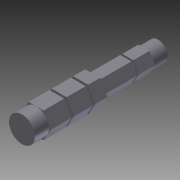
# Autodesk Inventor part: shaft - step down No. 1 - 0.5 hex
Saved by Autodesk Inventor 2012 (Build 160160000, 160)
## iProperties
Created: 2012-02-05
Part Number: shaft - step down No. 1 - 0.5 hex
Material: Steel
Document SubType Name: Modeling
Designer: Antonella Wilby
Mass: 56.1486 g
Surface Area: 25.2544 cm^2
Volume: 7.15269 cm^3
Density: 7.85 g/cm^3
Author: Antonella Wilby
Autodesk Inventor part; units mm, degrees
sketch "Sketch1" plane through (0, 0, 0) normal (0, 0, 1) x (1, 0, 0)
  line L0 (-10.3063, 0) -> (10.3063, 0) projected
  line L1 (0, -8.9256) -> (0, 8.9256) projected
  line L2 (3.6808, 6.3754) -> (7.3617, 0)
  line L3 (7.3617, 0) -> (3.6808, -6.3754)
  line L4 (3.6808, -6.3754) -> (-3.6808, -6.3754)
  line L5 (-3.6808, -6.3754) -> (-7.3617, 0)
  line L6 (-7.3617, 0) -> (-3.6808, 6.3754)
  line L7 (-3.6808, 6.3754) -> (3.6808, 6.3754)
  point P0 (0, 0)
  point P1 (0, 0)
  point P2 (0, 6.3754)
  dimension "d0" = 12.7508
  constraints: 12 end point, 1 coincident, 1 midpoint, 1 vertical alignment, 13 other
  measures "d0" distance between parallel lines of L7 L4
extrude "Base" add sketch "Sketch1" along normal mid plane 67.3354
sketch "Sketch2" plane through (0, 0, 33.6677) normal (0, 0, 1) x (1, 0, 0)
  line L0 (7.3617, 0) -> (3.6808, -6.3754) projected
  line L1 (3.6808, 6.3754) -> (7.3617, 0) projected
  line L2 (-3.6808, 6.3754) -> (3.6808, 6.3754) projected
  line L3 (-7.3617, 0) -> (-3.6808, 6.3754) projected
  line L4 (-3.6808, -6.3754) -> (-7.3617, 0) projected
  line L5 (3.6808, -6.3754) -> (-3.6808, -6.3754) projected
  circle A0 centre (0, 0) radius 6.3754
  constraints: 1 centre point, 1 coincident, 1 tangent
extrude "Bearing Fit" cut sketch "Sketch2" against normal blind 6.985 contours L0 A0 L1 | L0 L5 A0 | A0 L2 L1 | L5 L4 A0 | A0 L3 L2 | L4 L3 A0
mirror "Mirror1" about plane through (0, 0, 0) normal (0, 0, 1) of "Bearing Fit"
sketch "Sketch4" plane through (0, 0, -33.6677) normal (0, 0, -1) x (-1, 0, 0)
  circle A0 centre (0, 0) radius 6.3754 projected
  circle A1 centre (0, 0) radius 4.7625
  dimension "d7" = 9.525
  constraints: 1 centre point, 1 coincident
  measures "d7" diameter of A1
extrude "Extrusion4" cut sketch "Sketch4" against normal up to surface (6.985 mm away)
sketch "Sketch5" plane through (3.6808, 6.3754, -26.6827) normal (0, 0, -1) x (-1, 0, 0)
  line L0 (7.3617, 0) -> (11.0425, -6.3754) projected
  line L1 (0, 0) -> (7.3617, 0) projected
  line L2 (-3.6808, -6.3754) -> (0, 0) projected
  line L3 (0, -12.7508) -> (-3.6808, -6.3754) projected
  line L4 (7.3617, -12.7508) -> (0, -12.7508) projected
  line L5 (11.0425, -6.3754) -> (7.3617, -12.7508) projected
  line L6 (6.4305, -1.6129) -> (9.1801, -6.3754)
  line L7 (9.1801, -6.3754) -> (6.4305, -11.1379)
  line L8 (6.4305, -11.1379) -> (0.9312, -11.1379)
  line L9 (0.9312, -11.1379) -> (-1.8184, -6.3754)
  line L10 (-1.8184, -6.3754) -> (0.9312, -1.6129)
  line L11 (0.9312, -1.6129) -> (6.4305, -1.6129)
  dimension "d10" = 9.525
  constraints: 12 end point, 5 other
  measures "d10" distance between parallel lines of L11 L8
extrude ".375 step down" cut sketch "Sketch5" against normal blind 25.4
ref_plane "Work Plane1" through (0, 0, 15.2527) normal (0, 0, 1) x (1, 0, 0)
sketch "Sketch6" plane through (0, 0, 15.2527) normal (0, 0, 1) x (1, 0, 0)
  line L0 (-3.6808, 6.3754) -> (0, 6.3754) projected
  line L1 (-5.5213, 3.1877) -> (-3.6808, 6.3754) projected
  line L2 (3.6808, 6.3754) -> (5.5213, 3.1877) projected
  line L3 (0, 6.3754) -> (3.6808, 6.3754) projected
  line L4 (5.5213, 3.1877) -> (7.3617, 0) projected
  line L5 (7.3617, 0) -> (5.5213, -3.1877) projected
  line L6 (5.5213, -3.1877) -> (3.6808, -6.3754) projected
  line L7 (0, -6.3754) -> (-3.6808, -6.3754) projected
  line L8 (-3.6808, -6.3754) -> (-5.5213, -3.1877) projected
  line L9 (3.6808, -6.3754) -> (0, -6.3754) projected
  line L10 (-7.3617, 0) -> (-5.5213, 3.1877) projected
  line L11 (-5.5213, -3.1877) -> (-7.3617, 0) projected
  circle A0 centre (0, 0) radius 5.0292
  point P0 (0, 0)
  dimension "d14" = 10.0584
  constraints: 1 centre point, 1 coincident
  measures "d14" diameter of A0
extrude "Extrusion6" cut sketch "Sketch6" along normal blind 1.1684
ref_plane "Work Plane2" through (0, 0, 5.7785) normal (0, 0, 1) x (1, 0, 0)
sketch "Sketch7" plane through (0, 0, 5.7785) normal (0, 0, 1) x (1, 0, 0)
  line L0 (0, 6.3754) -> (3.6808, 6.3754) projected
  line L1 (3.6808, 6.3754) -> (5.5213, 3.1877) projected
  line L2 (5.5213, 3.1877) -> (7.3617, 0) projected
  line L3 (7.3617, 0) -> (5.5213, -3.1877) projected
  line L4 (5.5213, -3.1877) -> (3.6808, -6.3754) projected
  line L5 (3.6808, -6.3754) -> (0, -6.3754) projected
  line L6 (0, -6.3754) -> (-3.6808, -6.3754) projected
  line L7 (-3.6808, -6.3754) -> (-5.5213, -3.1877) projected
  line L8 (-7.3617, 0) -> (-5.5213, 3.1877) projected
  line L9 (-5.5213, 3.1877) -> (-3.6808, 6.3754) projected
  line L10 (-3.6808, 6.3754) -> (0, 6.3754) projected
  circle A0 centre (0, 0) radius 5.0292
  circle A1 centre (0, 0) radius 7.3617
  point P0 (0, 0)
  dimension "d18" = 10.0584
  constraints: 2 coincident, 1 centre point, 3 other
  measures "d18" diameter of A0
extrude "Extrusion7" cut sketch "Sketch7" against normal blind 1.1684
ref_plane "Work Plane3" through (0, 0, -18.7071) normal (0, 0, 1) x (1, 0, 0)
sketch "Sketch8" plane through (0, 0, -18.7071) normal (0, 0, 1) x (1, 0, 0)
  circle A0 centre (0, 0) radius 3.8481
  line L0 (-2.7496, 4.7625) -> (2.7496, 4.7625) projected
  line L1 (-5.4993, 0) -> (-2.7496, 4.7625) projected
  circle A1 centre (0, 0) radius 5.4993
  point P0 (0, 0)
  dimension "d22" = 7.6962
  constraints: 2 coincident, 1 centre point, 3 other
  measures "d22" diameter of A0
extrude "Extrusion8" cut sketch "Sketch8" along normal blind 0.9906
body "Solid1"
